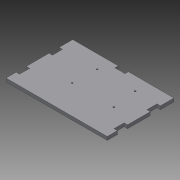
# Autodesk Inventor part: Controller_Base
Saved by Autodesk Inventor 2014 (Build 180170000, 170)
## iProperties
Created: 2014-11-10
Part Number: Controller_Base
Material: Generic
Document SubType Name: Modeling
Designer: ThatOtherGuy
Density: 1 g/cm^3
Appearance: Default
Author: ThatOtherGuy
Autodesk Inventor part; units mm, degrees
ref_plane "YZ Plane" through (0, 0, 0) normal (1, 0, 0) x (0, 1, 0)
ref_plane "XZ Plane" through (0, 0, 0) normal (0, 1, 0) x (-1, 0, 0)
ref_plane "XY Plane" through (0, 0, 0) normal (0, 0, 1) x (1, 0, 0)
sketch "Sketch1" plane through (0, 0, 0) normal (0, 0, 1) x (1, 0, 0)
  line L0 (0, 0) -> (200, 0)
  line L1 (200, 0) -> (200, 125)
  line L2 (200, 125) -> (0, 125)
  line L3 (0, 125) -> (0, 0)
  dimension "d23" = 200
  dimension "d24" = 125
  constraints: 8 end point, 2 parallel, 1 horizontal, 1 perpendicular
  measures "d23" distance of L1.end L2.end
  measures "d24" distance of L0.end L1.end
extrude "Extrusion1" add sketch "Sketch1" along normal blind 6.731
sketch "Sketch2" plane through (0, 0, 6.731) normal (0, 0, 1) x (1, 0, 0)
  line L0 (75.07, 105) -> (150, 105) construction
  line L1 (150, 105) -> (156.35, 105) construction
  line L2 (156.35, 105) -> (156.35, 56.74) construction
  line L3 (156.35, 56.74) -> (73.8, 56.74) construction
  line L4 (73.8, 56.74) -> (73.8, 105) construction
  line L5 (73.8, 105) -> (75.07, 105) construction
  line L6 (200, 0) -> (200, 125) projected
  line L7 (200, 125) -> (0, 125) projected
  dimension "d7" = 1.27
  dimension "d8" = 74.93
  dimension "d9" = 48.26
  dimension "d10" = 82.55
  dimension "d32" = 20
  dimension "d33" = 50
  constraints: 12 end point, 2 collinear, 2 parallel, 1 horizontal, 1 perpendicular
  measures "d7" distance of L4.end L0.start
  measures "d8" distance of L0.start L0.end
  measures "d9" distance of L3.end L4.end
  measures "d10" distance of L2.end L3.end
  measures "d32" distance from line of L7 L0.end
  measures "d33" distance from line of L6 L0.end
hole "Hole1" at (75.07, 105, 6.731) at (73.8, 56.74, 6.731) at (156.35, 56.74, 6.731) at (150, 105, 6.731) direction (0, 0, -1) diameter 3.176 end through all
sketch "Sketch3" plane through (0, 0, 6.731) normal (0, 0, 1) x (1, 0, 0)
  line L0 (200, 0) -> (200, 125) projected
  line L1 (0, 125) -> (0, 0) projected
  line L2 (0, 40) -> (6.731, 40)
  line L3 (6.731, 40) -> (6.731, 20)
  line L4 (6.731, 20) -> (0, 20)
  line L5 (0, 20) -> (0, 40)
  line L6 (200, 20) -> (193.269, 20)
  line L7 (193.269, 20) -> (193.269, 40)
  line L8 (193.269, 40) -> (200, 40)
  line L9 (200, 40) -> (200, 20)
  line L10 (0, 0) -> (200, 0) projected
  line L11 (0, 105) -> (6.731, 105)
  line L12 (6.731, 105) -> (6.731, 85)
  line L13 (6.731, 85) -> (0, 85)
  line L14 (0, 85) -> (0, 105)
  line L15 (200, 105) -> (193.269, 105)
  line L16 (193.269, 105) -> (193.269, 85)
  line L17 (193.269, 85) -> (200, 85)
  line L18 (200, 85) -> (200, 105)
  line L19 (90, 0) -> (110, 0)
  line L20 (110, 0) -> (110, 6.731)
  line L21 (110, 6.731) -> (90, 6.731)
  line L22 (90, 6.731) -> (90, 0)
  line L23 (200, 125) -> (0, 125) projected
  point P0 (100, 6.731)
  point P1 (100, 0)
  dimension "d19" = 6.731
  dimension "d20" = 20
  dimension "d25" = 20
  dimension "d28" = 20
  constraints: 40 end point, 10 parallel, 7 equal length, 5 horizontal, 5 perpendicular, 5 point on line, 3 collinear, 2 midpoint, 1 vertical alignment
  measures "d19" distance of L7.end L8.end
  measures "d20" distance of L2.end L3.end
  measures "d25" distance between parallel lines of L4 L10
  measures "d28" distance between parallel lines of L23 L11
extrude "Tabs" cut sketch "Sketch3" against normal up to next contours L6 L7 L8 L0 | L17 L16 L15 L0 | L1 L2 L3 L4 | L1 L11 L12 L13
sketch "Sketch4" plane through (0, 0, 6.731) normal (0, 0, 1) x (1, 0, 0)
  line L0 (0, 105) -> (6.731, 105) projected
  line L1 (0, 125) -> (90, 125)
  line L2 (90, 125) -> (90, 131.731)
  line L3 (90, 131.731) -> (0, 131.731)
  line L4 (0, 131.731) -> (0, 125)
  line L5 (200, 125) -> (110, 125)
  line L6 (110, 125) -> (110, 131.731)
  line L7 (110, 131.731) -> (200, 131.731)
  line L8 (200, 131.731) -> (200, 125)
  dimension "d29" = 20
  constraints: 16 end point, 4 parallel, 3 equal length, 2 horizontal, 2 perpendicular
  measures "d29" distance between parallel lines of L2 L6
extrude "Extrusion3" add sketch "Sketch4" against normal blind 6.731
equation "\"d0\" = THICKB"
equation "\"d19\" = THICKB"
equation "\"d21\" = THICKB"
equation "\"d30\" = THICKB"
equation "\"THICKA\" = 3.175"
equation "\"THICKB\" = 6.731"
equation "\"THICKC\" = 12.7"
equation "\"THICKPLY\" = 5"
equation "\"MAGDIA\" = 9.5"
equation "\"BALLDIA\" = 12"
body "Solid1"
